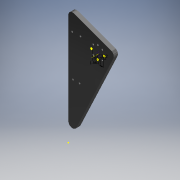
# Autodesk Inventor part: Triangle axle slide connector
Saved by Autodesk Inventor 2019 (Build 230136000, 136)
## iProperties
Part Number: Triangle axle slide connector
Material: Generic
Document SubType Name: Modeling
Designer: Delta
Appearance: Default
Author: Delta
Autodesk Inventor part; units mm, degrees
ref_plane "YZ Plane" through (0, 0, 0) normal (1, 0, 0) x (0, 1, 0)
ref_plane "XZ Plane" through (0, 0, 0) normal (0, 1, 0) x (-1, 0, 0)
ref_plane "XY Plane" through (0, 0, 0) normal (0, 0, 1) x (1, 0, 0)
sketch "Sketch1" plane through (0, 0, 0) normal (0, 0, 1) x (1, 0, 0)
  line L0 (0, 0) -> (0, 177.8)
  line L1 (0, 0) -> (53.8815, 0) construction
  line L2 (0, 177.8) -> (71.6046, 151.7381)
  line L3 (0, 177.8) -> (76.2, 177.8) construction
  line L4 (71.6046, 151.7381) -> (0, 0)
  dimension "d0" = 177.8
  dimension "d19" = 76.2
  dimension "d20" = 20
  constraints: 10 end point, 2 horizontal, 1 equal length, 1 vertical
  measures "d0" distance of L0.start L0.end
  measures "d19" distance of L0.end L2.end
  measures "d20" angle of L2 L3
extrude "Extrusion1" add sketch "Sketch1" along normal blind 6.35
fillet "Fillet1" radius 6.35 2 edges at (0, 177.8, 3.175) (0, 0, 3.175)
fillet "Fillet4" radius 6.35 1 edges at (71.6046, 151.7381, 3.175)
sketch "Sketch8" plane through (0, 0, 0) normal (0, 0, -1) x (-1, 0, 0)
  circle A0 centre (-44.8051, 141.6803) radius 2.54
  circle A1 centre (-44.8051, 151.4593) radius 1.3589
  circle A2 centre (-51.7199, 148.5951) radius 1.3589
  circle A3 centre (-54.5841, 141.6803) radius 1.3589
  circle A4 centre (-51.7199, 134.7655) radius 1.3589
  circle A5 centre (-44.8051, 131.9013) radius 1.3589
  circle A6 centre (-37.8903, 134.7655) radius 1.3589
  circle A7 centre (-35.0261, 141.6803) radius 1.3589
  circle A8 centre (-37.8903, 148.5951) radius 1.3589
  point P0 (0, 0)
  dimension "d60" = 5.08
  dimension "d61" = 2.7178
  dimension "d62" = 9.779
  dimension "d65" = 360
  constraints: 9 centre point, 17 other
  measures "d60" diameter of A0
  measures "d61" diameter of A1
  measures "d62" distance of A1.centre A0.centre
extrude "Extrusion7" cut sketch "Sketch8" against normal blind 25.4 contours A1 | A2 | A3 | A4 | A5 | A6 | A7 | A8
sketch "Sketch9" plane through (0, 0, 6.35) normal (0, 0, 1) x (1, 0, 0)
  circle A0 centre (35.0261, 141.6803) radius 1.3589 projected
  circle A1 centre (54.5841, 141.6803) radius 1.3589 projected
  circle A2 centre (44.8051, 131.9013) radius 1.3589 projected
  point P0 (0, 0)
  point P1 (46.164, 140.3214)
  dimension "d69" = 16.8402
  dimension "d70" = 8.4201
  dimension "d71" = 8.4201
  measures "d70" horizontal distance of A1.centre point (46.164, 140.321)
  measures "d71" vertical distance of point (46.164, 140.321) A2.centre
sketch "Sketch10" plane through (0, 0, 6.35) normal (0, 0, 1) x (1, 0, 0)
  circle A0 centre (18.3336, 149.503) radius 1.3589
  circle A1 centre (5.61, 149.2894) radius 1.3589
  line L0 (65.0627, 154.1191) -> (8.5218, 174.6983) projected
  point P0 (0, 0)
  dimension "d72" = 2.7178
  dimension "d73" = 2.7178
  dimension "d74" = 20.32
  dimension "d83" = 10.0076
  constraints: 2 centre point
  measures "d72" diameter of A0
  measures "d73" diameter of A1
  measures "d74" distance from line of L0 A0.centre
extrude "Extrusion8" cut sketch "Sketch10" against normal blind 25.4
sketch "Sketch11" plane through (0, 0, 6.35) normal (0, 0, 1) x (1, 0, 0)
  circle A0 centre (16.9311, 86.7557) radius 1.3589
  circle A1 centre (6.9237, 86.8299) radius 1.3589
  arc A2 (0, 28.3357) -> (12.0927, 25.6258) centre (6.35, 28.3357) ccw projected
  point P0 (0, 0)
  dimension "d77" = 2.7178
  dimension "d78" = 2.7178
  dimension "d79" = 58.42
  dimension "d82" = 10.0076
  constraints: 2 centre point
  measures "d77" diameter of A0
  measures "d78" diameter of A1
  measures "d79" vertical distance of A2.centre A0.centre
  measures "d82" distance of A1.centre A0.centre
extrude "Extrusion9" cut sketch "Sketch11" against normal blind 17.17
equation "\"d70\" = 0.5 * d69"
equation "\"d71\" = d70"
body "Solid1"
